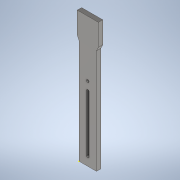
# Autodesk Inventor part: Part2
Saved by Autodesk Inventor 2021 (Build 250183000, 183)
## iProperties
Created: 2021-06-26
Part Number: Part2
Material: Steel, Cast
Document SubType Name: Modeling
Designer: VK
Density: 7.85 g/cm^3
Appearance: Semi-Polished
Author: VK
Autodesk Inventor part; units mm, degrees
ref_plane "YZ Plane" through (0, 0, 0) normal (1, 0, 0) x (0, 1, 0)
ref_plane "XZ Plane" through (0, 0, 0) normal (0, 1, 0) x (-1, 0, 0)
ref_plane "XY Plane" through (0, 0, 0) normal (0, 0, 1) x (1, 0, 0)
sketch "Sketch1" plane through (0, 0, 0) normal (0, 0, 1) x (1, 0, 0)
  line L0 (0, 0) -> (20, 0)
  line L1 (20, 0) -> (20, 120)
  line L2 (0, 0) -> (0, 120)
  line L3 (0, 0) -> (120, 0) construction
  line L4 (20, 120) -> (22.1131, 124.5315)
  line L5 (20, 120) -> (25, 120) construction
  line L6 (0, 120) -> (-2.1131, 124.5315)
  line L7 (-2.1131, 124.5315) -> (-2.1131, 149.5315)
  line L8 (-2.1131, 149.5315) -> (22.1131, 149.5315)
  line L9 (22.1131, 149.5315) -> (22.1131, 124.5315)
  dimension "d0" = 20
  dimension "d1" = 120
  dimension "d2" = 90
  dimension "d3" = 120
  dimension "d4" = 90
  dimension "d5" = 5
  dimension "d6" = 65
  dimension "d7" = 5
  dimension "d8" = 25
  constraints: 20 end point, 3 horizontal, 3 perpendicular, 2 equal length, 2 vertical
  measures "d0" distance of L0.start L0.end
  measures "d1" distance of L0.end L1.end
  measures "d2" angle of L1 L0
  measures "d3" distance of L0.start L2.end
  measures "d4" angle of L3 L2
  measures "d5" distance of L1.end L4.end
  measures "d6" angle of L5 L4
  measures "d7" distance of L2.end L6.end
  measures "d8" distance of L6.end L7.end
extrude "Extrusion1" add sketch "Sketch1" along normal blind 5
sketch "Sketch2" plane through (0, 0, 5) normal (0, 0, 1) x (1, 0, 0)
  point P0 (0, 0)
  point P1 (10, 10)
hole "Hole1" at (10, 10, 5) direction (0, 0, -1) diameter 3 end through all
sketch "Sketch3" plane through (0, 0, 5) normal (0, 0, 1) x (1, 0, 0)
  point P0 (0, 0)
sketch "Sketch4" plane through (0, 0, 5) normal (0, 0, 1) x (1, 0, 0)
  point P0 (0, 0)
  point P1 (10, 75)
hole "Hole2" at (10, 75, 5) direction (0, 0, -1) diameter 3 end through all
sketch "Sketch5" plane through (0, 0, 5) normal (0, 0, 1) x (1, 0, 0)
  circle A0 centre (10, 10) radius 1.5 projected
  line L0 (11.4716, 74.9905) -> (8.5, 74.9905)
  line L1 (8.5, 74.9905) -> (8.5, 10)
  line L2 (8.5, 10) -> (11.4716, 10)
  line L3 (11.4716, 10) -> (11.4716, 74.9905)
  point P0 (0, 0)
  constraints: 8 end point, 2 parallel, 1 horizontal, 1 horizontal alignment, 1 perpendicular, 1 other
extrude "Extrusion2" cut sketch "Sketch5" against normal blind 10 contours L1 L0 L3 A0 | A0 L3 L2 picked at (9.5055, 10.1215)
sketch "Sketch6" plane through (0, 0, 5) normal (0, 0, 1) x (1, 0, 0)
  point P0 (0, 0)
  point P1 (10, 85)
hole "Hole3" at (10, 85, 5) direction (0, 0, -1) diameter 3 end through all
sketch "Sketch8" plane through (0, 0, 0) normal (0, 0, -1) x (-1, 0, 0)
  point P0 (0, 0)
  point P1 (-10, -8)
hole "Hole4" at (10, -8, 0) direction (0, 0, 1) diameter 3 end through all
sketch "Sketch10" plane through (0, 0, 5) normal (0, 0, 1) x (1, 0, 0)
  line L0 (22.1131, 124.5315) -> (22.1131, 149.5315) projected
  line L1 (-2.1131, 149.5315) -> (-2.1131, 124.5315) projected
  point P0 (0, 0)
  dimension "d45" = 24.2262
  measures "d45" distance between parallel lines of L0 L1
sketch "Sketch11" plane through (0, 0, 5) normal (0, 0, 1) x (1, 0, 0)
  point P0 (0, 0)
sketch "Sketch12" plane through (0, 0, 5) normal (0, 0, 1) x (1, 0, 0)
  point P0 (0, 0)
sketch "Sketch13" plane through (0, 0, 5) normal (0, 0, 1) x (1, 0, 0)
  point P0 (0, 0)
body "Solid1"
